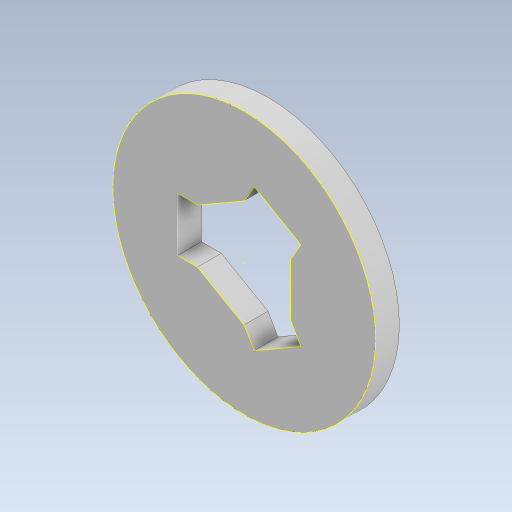
# Autodesk Inventor part: 2GTbase
Saved by Autodesk Inventor 2023 (Build 270158000, 158)
## iProperties
Created: 2023-05-15
Part Number: 2GTbase
Material: 一般
Document SubType Name: Modeling
Designer: Johnny Jou
Density: 1 g/cm^3
Appearance: 預設
Author: Johnny Jou
Autodesk Inventor part; units mm, degrees
ref_plane "YZ Plane" through (0, 0, 0) normal (1, 0, 0) x (0, 1, 0)
ref_plane "XZ Plane" through (0, 0, 0) normal (0, 1, 0) x (-1, 0, 0)
ref_plane "XY Plane" through (0, 0, 0) normal (0, 0, 1) x (1, 0, 0)
sketch "草圖1" plane through (0, 0, 0) normal (0, 0, 1) x (1, 0, 0)
  line L0 (5.85, -3.3775) -> (0, -6.755)
  line L1 (5.85, 3.3775) -> (5.85, -3.3775)
  line L2 (0, 6.755) -> (5.85, 3.3775)
  line L3 (-5.85, 3.3775) -> (0, 6.755)
  line L4 (-5.85, -3.3775) -> (-5.85, 3.3775)
  line L5 (0, -6.755) -> (-5.85, -3.3775)
  line L6 (-5.85, 3.3775) -> (0, 6.755)
  line L7 (0, 6.755) -> (5.85, 3.3775)
  line L8 (0, 6.755) -> (5.85, 3.3775)
  line L9 (5.85, 3.3775) -> (7.1, 5.5426)
  line L10 (7.1, 5.5426) -> (1.25, 8.9201)
  line L11 (1.25, 8.9201) -> (0, 6.755)
  line L12 (-5.85, -3.3775) -> (-5.85, 3.3775)
  line L13 (-5.85, 3.3775) -> (-8.35, 3.3775)
  line L14 (-8.35, 3.3775) -> (-8.35, -3.3775)
  line L15 (-8.35, -3.3775) -> (-5.85, -3.3775)
  line L16 (5.85, -3.3775) -> (0, -6.755)
  line L17 (0, -6.755) -> (1.25, -8.9201)
  line L18 (1.25, -8.9201) -> (7.1, -5.5426)
  line L19 (7.1, -5.5426) -> (5.85, -3.3775)
  circle A0 centre (0, 0) radius 16.5
  point P0 (0, -6.755)
  dimension "d2" = 2.5
  dimension "d3" = 360
  dimension "d4" = 33
  constraints: 40 end point, 9 equal length, 2 coincident, 1 centre point, 1 perpendicular, 25 other
  measures "d2" distance of L9.start L9.end
  measures "d4" diameter of A0
extrude "擠出1" add sketch "草圖1" along normal blind 3
sketch "草圖2" plane through (0, 0, 3) normal (0, 0, 1) x (1, 0, 0)
  circle A0 centre (0, 0) radius 16.5 projected
  line L0 (0, 6.755) -> (1.25, 8.9201) projected
  line L1 (1.25, 8.9201) -> (7.1, 5.5426) projected
  line L2 (7.1, 5.5426) -> (5.85, 3.3775) projected
  line L3 (5.85, 3.3775) -> (5.85, -3.3775) projected
  line L4 (5.85, -3.3775) -> (7.1, -5.5426) projected
  line L5 (7.1, -5.5426) -> (1.25, -8.9201) projected
  line L6 (1.25, -8.9201) -> (0, -6.755) projected
  line L7 (0, -6.755) -> (-5.85, -3.3775) projected
  line L8 (-5.85, -3.3775) -> (-8.35, -3.3775) projected
  line L9 (-8.35, -3.3775) -> (-8.35, 3.3775) projected
  line L10 (-8.35, 3.3775) -> (-5.85, 3.3775) projected
  line L11 (-5.85, 3.3775) -> (0, 6.755) projected
